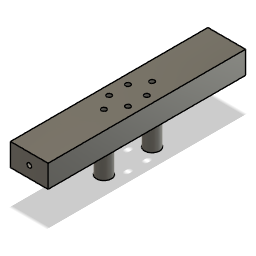
Assemply v7 (Autodesk Fusion 360 archive; units mm, degrees)
design "GPS+hinge stand"
Autodesk Fusion 360 part; units mm, degrees
(part 1 of 5)
sketch "Sketch1" plane through (0, 0, 0) normal (0, 0, 1) x (1, 0, 0)
  line L0 (0, 0) -> (25, 0)
  line L1 (25, 0) -> (25, 15)
  line L2 (25, 15) -> (0, 15)
  line L3 (0, 15) -> (0, 0)
  dimension "d1" = 25
  dimension "d2" = 15
  constraint horizontal L0
  constraint vertical L1
  constraint horizontal L2
  constraint vertical L3
  constraint coincident L0.start L3.end
  measures "d1" distance of L0.start L0.end
  measures "d2" distance of L0.start L2.end
extrude "Extrude1" add sketch "Sketch1" along normal blind 131.11
sketch "Sketch2" plane through (0, 0, 131.11) normal (0, 0, 1) x (1, 0, 0)
  line L0 (0, 15) -> (0, 0)
  line L1 (0, 0) -> (25, 0)
  line L2 (25, 0) -> (25, 15)
  line L3 (25, 15) -> (0, 15)
  circle A0 centre (12.5, 7.5) radius 1.5
  dimension "d5" = 3
  measures "d5" diameter of A0
extrude "Extrude2" cut sketch "Sketch2" against normal blind 180 contours A0
sketch "Sketch3" plane through (0, 15, 0) normal (0, 1, 0) x (-1, 0, 0)
  line L0 (-25, 0) -> (0, 0)
  line L1 (0, 0) -> (0, 131.11)
  line L2 (0, 131.11) -> (-25, 131.11)
  line L3 (-25, 131.11) -> (-25, 0)
  circle A0 centre (-12.5, 49.555) radius 1.6
  circle A1 centre (-12.5, 81.555) radius 1.6
  dimension "d8" = 3.2
  dimension "d24" = 3.2
  measures "d8" diameter of A0
  measures "d24" diameter of A1
extrude "Extrude3" cut sketch "Sketch3" against normal blind 51 contours A0 | A1
sketch "Sketch4" plane through (0, 15, 0) normal (0, 1, 0) x (-1, 0, 0)
  circle A0 centre (-12.5, 81.555) radius 1.6
  circle A1 centre (-12.5, 49.555) radius 1.6
  line L0 (-25, 0) -> (0, 0)
  line L1 (0, 0) -> (0, 131.11)
  line L2 (0, 131.11) -> (-25, 131.11)
  line L3 (-25, 131.11) -> (-25, 0)
  line L4 (-25, 78.055) -> (0, 78.055)
  line L5 (0, 78.055) -> (0, 53.055)
  line L6 (0, 53.055) -> (-25, 53.055)
  line L7 (-25, 53.055) -> (-25, 78.055)
  line L8 (-25, 78.055) -> (0, 53.055) construction
  line L9 (0, 78.055) -> (-25, 53.055) construction
  point P0 (-12.5, 65.555)
  dimension "d12" = 25
  dimension "d13" = 25
  constraint horizontal L4
  constraint perpendicular L4 L5
  constraint parallel L4 L6
  constraint parallel L5 L7
  constraint coincident L8 P0
  constraint coincident L9 P0
  measures "d12" distance of L5.end L6.end
  measures "d13" distance of L4.end L5.end
sketch "Sketch6" plane through (0, 0, 0) normal (0, -1, 0) x (1, 0, 0)
  circle A0 centre (12.5, 81.555) radius 1.6
  circle A1 centre (12.5, 49.555) radius 1.6
  line L0 (0, 0) -> (25, 0)
  line L1 (25, 0) -> (25, 131.11)
  line L2 (25, 131.11) -> (0, 131.11)
  line L3 (0, 131.11) -> (0, 0)
  circle A2 centre (12.5, 81.555) radius 5
  circle A3 centre (12.5, 49.555) radius 5
  dimension "d20" = 10
  dimension "d21" = 10
  constraint concentric A0 A2
  constraint concentric A1 A3
  measures "d20" diameter of A2
  measures "d21" diameter of A3
extrude "Extrude6" add sketch "Sketch6" along normal blind 22.5 contours A2 | A3
sketch "Sketch7" plane through (0, 15, 0) normal (0, 1, 0) x (-1, 0, 0)
  circle A0 centre (-12.5, 81.555) radius 1.6
  circle A1 centre (-12.5, 49.555) radius 1.6
  line L0 (-25, 0) -> (0, 0)
  line L1 (0, 0) -> (0, 131.11)
  line L2 (0, 131.11) -> (-25, 131.11)
  line L3 (-25, 131.11) -> (-25, 0)
  line L4 (-25, 53.055) -> (0, 53.055)
  line L5 (0, 53.055) -> (0, 78.055)
  line L6 (0, 78.055) -> (-25, 78.055)
  line L7 (-25, 78.055) -> (-25, 53.055)
  circle A2 centre (-6.25, 59.305) radius 1.6
  circle A3 centre (-6.25, 71.805) radius 1.6
  line L8 (-12.5, 65.555) -> (-12.5, 69)
  circle A4 centre (-18.75, 59.305) radius 1.6
  circle A5 centre (-18.75, 71.805) radius 1.6
  point P0 (-12.5, 65.555)
  dimension "d25" = 25
  dimension "d26" = 25
  dimension "d27" = 3.2
  dimension "d28" = 6.25
  dimension "d29" = 6.25
  dimension "d30" = 3.2
  dimension "d31" = 12.5
  constraint horizontal L4
  constraint perpendicular L4 L5
  constraint parallel L4 L6
  constraint parallel L5 L7
  constraint coincident P0 L8.start
  constraint parallel L5 L8
  constraint symmetric A2 L8 A4
  constraint symmetric A3 L8 A5
  measures "d25" distance of L5.end L6.end
  measures "d26" distance of L4.end L5.end
  measures "d27" diameter of A2
  measures "d28" horizontal distance of P0 A2.centre
  measures "d29" distance of L4 A2.centre
  measures "d30" diameter of A3
  measures "d31" distance of A2.centre A3.centre
extrude "Extrude7" cut sketch "Sketch7" against normal blind 17 contours A2 | A3 | A4 | A5
fillet "Fillet1" radius 7.5 2 edges at (7.8384, 0, 83.3631) (7.8384, 0, 51.3631)
sketch "Sketch8" plane through (0, 0, 0) normal (0, -1, 0) x (1, 0, 0)
  arc A0 (4.6502, 59.2828) -> (0, 49.555) centre (12.5, 49.555) ccw
  arc A1 (6.9381, 60.7495) -> (4.6502, 59.2828) centre (6.25, 59.305) ccw
  arc A2 (18.0619, 60.7495) -> (6.9381, 60.7495) centre (12.5, 49.555) ccw
  arc A3 (20.3498, 59.2828) -> (18.0619, 60.7495) centre (18.75, 59.305) ccw
  arc A4 (25, 49.555) -> (20.3498, 59.2828) centre (12.5, 49.555) ccw
  line L0 (25, 49.555) -> (25, 81.555)
  arc A5 (20.3498, 71.8272) -> (25, 81.555) centre (12.5, 81.555) ccw
  arc A6 (18.0619, 70.3605) -> (20.3498, 71.8272) centre (18.75, 71.805) ccw
  arc A7 (6.9381, 70.3605) -> (18.0619, 70.3605) centre (12.5, 81.555) ccw
  arc A8 (4.6502, 71.8272) -> (6.9381, 70.3605) centre (6.25, 71.805) ccw
  arc A9 (0, 81.555) -> (4.6502, 71.8272) centre (12.5, 81.555) ccw
  line L1 (0, 81.555) -> (0, 49.555)
  circle A10 centre (6.25, 59.305) radius 3.5
  circle A11 centre (18.75, 59.305) radius 3.5
  circle A12 centre (6.25, 71.805) radius 3.5
  circle A13 centre (18.75, 71.805) radius 3.5
  dimension "d36" = 7
  dimension "d37" = 7
  dimension "d38" = 7
  dimension "d39" = 7
  constraint concentric A1 A10
  constraint concentric A3 A11
  constraint concentric A8 A12
  constraint concentric A6 A13
  measures "d36" diameter of A10
  measures "d37" diameter of A11
  measures "d38" diameter of A12
  measures "d39" diameter of A13
extrude "Extrude8" cut sketch "Sketch8" along normal blind 6 contours A0 A1 A2 A10 | A2 A3 A4 A11 | A7 A8 A9 A12 | A5 A6 A7 A13 picked at (6.5291, 58.7685) picked at (18.3538, 58.8458) picked at (6.5291, 72.3415) picked at (18.4982, 72.3568)
equation "d22 = 42.5 mm - 40 mm + 20 mm"
equation "d28 = 25 / 4 * 1 mm"
equation "d31 = 25 / 2 * 1 mm"

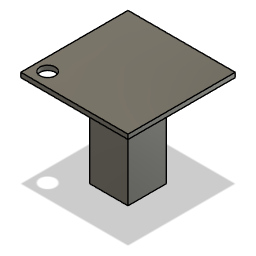
design "Gps mount"
Autodesk Fusion 360 part; units mm, degrees
sketch "Sketch1" plane through (0, 0, 0) normal (0, 1, 0) x (1, 0, 0)
  line L0 (0, 0) -> (25, 0)
  line L1 (25, 0) -> (25, -25)
  line L2 (25, -25) -> (0, -25)
  line L3 (0, -25) -> (0, 0)
  dimension "d1" = 25
  dimension "d2" = 25
  constraint horizontal L0
  constraint vertical L1
  constraint horizontal L2
  constraint vertical L3
  constraint coincident L0.start L3.end
  measures "d1" distance of L0.start L0.end
  measures "d2" distance of L0.start L2.end
extrude "Extrude1" add sketch "Sketch1" along normal blind 60
sketch "Sketch2" plane through (0, 60, 0) normal (0, 1, 0) x (-1, 0, 0)
  line L0 (0, 25) -> (-25, 25)
  line L1 (-25, 25) -> (-25, 0)
  line L2 (-25, 0) -> (0, 0)
  line L3 (0, 0) -> (0, 25)
  line L4 (-47.5, 47.5) -> (22.5, 47.5)
  line L5 (22.5, 47.5) -> (22.5, -22.5)
  line L6 (22.5, -22.5) -> (-47.5, -22.5)
  line L7 (-47.5, -22.5) -> (-47.5, 47.5)
  line L8 (-47.5, 47.5) -> (22.5, -22.5) construction
  line L9 (22.5, 47.5) -> (-47.5, -22.5) construction
  point P0 (-12.5, 12.5)
  dimension "d5" = 70
  dimension "d6" = 70
  constraint horizontal L4
  constraint perpendicular L4 L5
  constraint parallel L4 L6
  constraint parallel L5 L7
  constraint coincident L8 P0
  constraint coincident L9 P0
  measures "d5" distance of L5.end L6.end
  measures "d6" distance of L4.end L5.end
extrude "Extrude2" add sketch "Sketch2" along normal blind 3 contours L0 L1 L2 L3 | L4 L5 L6 L7
fillet "Fillet1" radius 10 4 edges at (12.5, 60, 25) (25, 60, 12.5) (0, 60, 12.5) (12.5, 60, 0)
sketch "Sketch3" plane through (0, 63, 0) normal (0, 1, 0) x (-1, 0, 0)
  line L0 (-47.5, -22.5) -> (22.5, -22.5)
  line L1 (22.5, -22.5) -> (22.5, 47.5)
  line L2 (22.5, 47.5) -> (-47.5, 47.5)
  line L3 (-47.5, 47.5) -> (-47.5, -22.5)
  circle A0 centre (14.2428, 38.2388) radius 5
  dimension "d11" = 10
  measures "d11" diameter of A0
extrude "Extrude3" cut sketch "Sketch3" against normal blind 30 contours A0
sketch "Sketch4" plane through (0, 0, 0) normal (0, 1, 0) x (1, 0, 0)
  line L0 (25, 0) -> (0, 0)
  line L1 (0, 0) -> (0, -25)
  line L2 (0, -25) -> (25, -25)
  line L3 (25, -25) -> (25, 0)
  circle A0 centre (18.75, -6.25) radius 1.5
  circle A1 centre (18.767, -18.75) radius 1.5
  circle A2 centre (6.25, -6.25) radius 1.5
  circle A3 centre (6.233, -18.75) radius 1.5
  point P0 (25, 0)
  point P1 (25, -25)
  dimension "d14" = 3
  dimension "d15" = 3
  dimension "d17" = 12.5
  dimension "d18" = 6.25
  constraint horizontal L0
  constraint vertical L1
  constraint horizontal L2
  constraint vertical L3
  constraint coincident L0 P0
  constraint coincident L2 P1
  measures "d14" diameter of A0
  measures "d15" diameter of A1
  measures "d17" vertical distance of A0.centre A1.centre
  measures "d18" distance of L2 A1.centre
extrude "Extrude4" cut sketch "Sketch4" along normal blind 7 contours A0 | A1 | A2 | A3
equation "d17 = 2.5 / 2 * 1 cm"
equation "d18 = 2.5 / 4 * 1 cm"

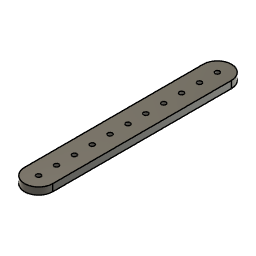
design "Camera arm 1"
Autodesk Fusion 360 part; units mm, degrees
sketch "Sketch1" plane through (0, 0, 0) normal (0, 1, 0) x (1, 0, 0)
  line L0 (20, 0) -> (20, -127)
  line L1 (0, -127) -> (0, 0)
  arc A0 (0, -127) -> (20, -127) centre (10, -127) ccw
  arc A1 (20, 0) -> (0, 0) centre (10, 0) ccw
  circle A2 centre (10, 0) radius 1.6
  circle A3 centre (10, -127) radius 1.6
  circle A4 centre (10, -114.3) radius 1.6
  circle A5 centre (10, -101.6) radius 1.6
  circle A6 centre (10, -88.9) radius 1.6
  circle A7 centre (10, -76.2) radius 1.6
  circle A8 centre (10, -63.5) radius 1.6
  circle A9 centre (10, -50.8) radius 1.6
  circle A10 centre (10, -38.1) radius 1.6
  circle A11 centre (10, -25.4) radius 1.6
  circle A12 centre (10, -12.7) radius 1.6
  dimension "d1" = 20
  dimension "d2" = 127
  dimension "d3" = 3.2
  dimension "d4" = 3.2
  dimension "d9" = 0
  dimension "d10" = 12.7
  constraint vertical L0
  constraint vertical L1
  constraint coincident L1.end A1.end
  constraint concentric A1 A2
  constraint concentric A0 A3
  measures "d1" distance of L1.end L0.start
  measures "d2" distance of L1.end L1.start
  measures "d3" diameter of A2
  measures "d4" diameter of A3
extrude "Extrude1" add sketch "Sketch1" along normal blind 5

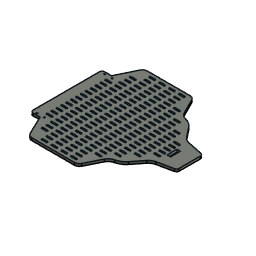
design "Electronics plate"
Autodesk Fusion 360 part; units mm, degrees
sketch "Sketch2" plane through (0, 0, 0) normal (0, 1, 0) x (1, 0, 0)
  line L0 (-228.4396, 191.0218) -> (-250, 146.0218)
  line L1 (-249.9865, 0) -> (-228.4396, -44.9718)
  line L2 (-128.4396, 191.0218) -> (-228.4396, 191.0218)
  line L3 (-228.4396, -44.9718) -> (-128.4396, -44.9718)
  line L4 (-105.9194, 146.05) -> (-128.4396, 191.0218)
  line L5 (-128.4396, -44.9718) -> (-105.9194, 0)
  line L6 (-138.6977, 71.525) -> (-143.6977, 71.525)
  line L7 (-148.6977, 74.525) -> (-138.6977, 74.525)
  arc A0 (-138.6977, 71.525) -> (-138.6977, 74.525) centre (-138.6977, 73.025) ccw
  arc A1 (-148.6977, 74.525) -> (-148.6977, 71.525) centre (-148.6977, 73.025) ccw
  line L8 (-148.6977, 71.525) -> (-143.6977, 71.525)
  arc A2 (-208.6977, -35.475) -> (-208.6977, -38.475) centre (-208.6977, -36.975) ccw
  arc A3 (-198.6977, -38.475) -> (-198.6977, -35.475) centre (-198.6977, -36.975) ccw
  line L9 (-208.6977, -35.475) -> (-198.6977, -35.475)
  line L10 (-208.6977, -38.475) -> (-203.6977, -38.475)
  line L11 (-198.6977, -38.475) -> (-203.6977, -38.475)
  arc A4 (-188.6977, -35.475) -> (-188.6977, -38.475) centre (-188.6977, -36.975) ccw
  arc A5 (-178.6977, -38.475) -> (-178.6977, -35.475) centre (-178.6977, -36.975) ccw
  line L12 (-188.6977, -35.475) -> (-178.6977, -35.475)
  line L13 (-188.6977, -38.475) -> (-183.6977, -38.475)
  line L14 (-178.6977, -38.475) -> (-183.6977, -38.475)
  arc A6 (-168.6977, -35.475) -> (-168.6977, -38.475) centre (-168.6977, -36.975) ccw
  arc A7 (-158.6977, -38.475) -> (-158.6977, -35.475) centre (-158.6977, -36.975) ccw
  line L15 (-168.6977, -35.475) -> (-158.6977, -35.475)
  line L16 (-168.6977, -38.475) -> (-163.6977, -38.475)
  line L17 (-158.6977, -38.475) -> (-163.6977, -38.475)
  arc A8 (-148.6977, -35.475) -> (-148.6977, -38.475) centre (-148.6977, -36.975) ccw
  arc A9 (-138.6977, -38.475) -> (-138.6977, -35.475) centre (-138.6977, -36.975) ccw
  line L18 (-148.6977, -35.475) -> (-138.6977, -35.475)
  line L19 (-148.6977, -38.475) -> (-143.6977, -38.475)
  line L20 (-138.6977, -38.475) -> (-143.6977, -38.475)
  arc A10 (-208.6977, -25.475) -> (-208.6977, -28.475) centre (-208.6977, -26.975) ccw
  arc A11 (-198.6977, -28.475) -> (-198.6977, -25.475) centre (-198.6977, -26.975) ccw
  line L21 (-208.6977, -25.475) -> (-198.6977, -25.475)
  line L22 (-208.6977, -28.475) -> (-203.6977, -28.475)
  line L23 (-198.6977, -28.475) -> (-203.6977, -28.475)
  arc A12 (-188.6977, -25.475) -> (-188.6977, -28.475) centre (-188.6977, -26.975) ccw
  arc A13 (-178.6977, -28.475) -> (-178.6977, -25.475) centre (-178.6977, -26.975) ccw
  line L24 (-188.6977, -25.475) -> (-178.6977, -25.475)
  line L25 (-188.6977, -28.475) -> (-183.6977, -28.475)
  line L26 (-178.6977, -28.475) -> (-183.6977, -28.475)
  arc A14 (-168.6977, -25.475) -> (-168.6977, -28.475) centre (-168.6977, -26.975) ccw
  arc A15 (-158.6977, -28.475) -> (-158.6977, -25.475) centre (-158.6977, -26.975) ccw
  line L27 (-168.6977, -25.475) -> (-158.6977, -25.475)
  line L28 (-168.6977, -28.475) -> (-163.6977, -28.475)
  line L29 (-158.6977, -28.475) -> (-163.6977, -28.475)
  arc A16 (-148.6977, -25.475) -> (-148.6977, -28.475) centre (-148.6977, -26.975) ccw
  arc A17 (-138.6977, -28.475) -> (-138.6977, -25.475) centre (-138.6977, -26.975) ccw
  line L30 (-148.6977, -25.475) -> (-138.6977, -25.475)
  line L31 (-148.6977, -28.475) -> (-143.6977, -28.475)
  line L32 (-138.6977, -28.475) -> (-143.6977, -28.475)
  arc A18 (-228.6977, -15.475) -> (-228.6977, -18.475) centre (-228.6977, -16.975) ccw
  arc A19 (-218.6977, -18.475) -> (-218.6977, -15.475) centre (-218.6977, -16.975) ccw
  line L33 (-228.6977, -15.475) -> (-218.6977, -15.475)
  line L34 (-228.6977, -18.475) -> (-223.6977, -18.475)
  line L35 (-218.6977, -18.475) -> (-223.6977, -18.475)
  arc A20 (-208.6977, -15.475) -> (-208.6977, -18.475) centre (-208.6977, -16.975) ccw
  arc A21 (-198.6977, -18.475) -> (-198.6977, -15.475) centre (-198.6977, -16.975) ccw
  line L36 (-208.6977, -15.475) -> (-198.6977, -15.475)
  line L37 (-208.6977, -18.475) -> (-203.6977, -18.475)
  line L38 (-198.6977, -18.475) -> (-203.6977, -18.475)
  arc A22 (-188.6977, -15.475) -> (-188.6977, -18.475) centre (-188.6977, -16.975) ccw
  arc A23 (-178.6977, -18.475) -> (-178.6977, -15.475) centre (-178.6977, -16.975) ccw
  line L39 (-188.6977, -15.475) -> (-178.6977, -15.475)
  line L40 (-188.6977, -18.475) -> (-183.6977, -18.475)
  line L41 (-178.6977, -18.475) -> (-183.6977, -18.475)
  arc A24 (-168.6977, -15.475) -> (-168.6977, -18.475) centre (-168.6977, -16.975) ccw
  arc A25 (-158.6977, -18.475) -> (-158.6977, -15.475) centre (-158.6977, -16.975) ccw
  line L42 (-168.6977, -15.475) -> (-158.6977, -15.475)
  line L43 (-168.6977, -18.475) -> (-163.6977, -18.475)
  line L44 (-158.6977, -18.475) -> (-163.6977, -18.475)
  arc A26 (-148.6977, -15.475) -> (-148.6977, -18.475) centre (-148.6977, -16.975) ccw
  arc A27 (-138.6977, -18.475) -> (-138.6977, -15.475) centre (-138.6977, -16.975) ccw
  line L45 (-148.6977, -15.475) -> (-138.6977, -15.475)
  line L46 (-148.6977, -18.475) -> (-143.6977, -18.475)
  line L47 (-138.6977, -18.475) -> (-143.6977, -18.475)
  arc A28 (-228.6977, -5.475) -> (-228.6977, -8.475) centre (-228.6977, -6.975) ccw
  arc A29 (-218.6977, -8.475) -> (-218.6977, -5.475) centre (-218.6977, -6.975) ccw
  line L48 (-228.6977, -5.475) -> (-218.6977, -5.475)
  line L49 (-228.6977, -8.475) -> (-223.6977, -8.475)
  line L50 (-218.6977, -8.475) -> (-223.6977, -8.475)
  arc A30 (-208.6977, -5.475) -> (-208.6977, -8.475) centre (-208.6977, -6.975) ccw
  arc A31 (-198.6977, -8.475) -> (-198.6977, -5.475) centre (-198.6977, -6.975) ccw
  line L51 (-208.6977, -5.475) -> (-198.6977, -5.475)
  line L52 (-208.6977, -8.475) -> (-203.6977, -8.475)
  line L53 (-198.6977, -8.475) -> (-203.6977, -8.475)
  arc A32 (-188.6977, -5.475) -> (-188.6977, -8.475) centre (-188.6977, -6.975) ccw
  arc A33 (-178.6977, -8.475) -> (-178.6977, -5.475) centre (-178.6977, -6.975) ccw
  line L54 (-188.6977, -5.475) -> (-178.6977, -5.475)
  line L55 (-188.6977, -8.475) -> (-183.6977, -8.475)
  line L56 (-178.6977, -8.475) -> (-183.6977, -8.475)
  arc A34 (-168.6977, -5.475) -> (-168.6977, -8.475) centre (-168.6977, -6.975) ccw
  arc A35 (-158.6977, -8.475) -> (-158.6977, -5.475) centre (-158.6977, -6.975) ccw
  line L57 (-168.6977, -5.475) -> (-158.6977, -5.475)
  line L58 (-168.6977, -8.475) -> (-163.6977, -8.475)
  line L59 (-158.6977, -8.475) -> (-163.6977, -8.475)
  arc A36 (-148.6977, -5.475) -> (-148.6977, -8.475) centre (-148.6977, -6.975) ccw
  arc A37 (-138.6977, -8.475) -> (-138.6977, -5.475) centre (-138.6977, -6.975) ccw
  line L60 (-148.6977, -5.475) -> (-138.6977, -5.475)
  line L61 (-148.6977, -8.475) -> (-143.6977, -8.475)
  line L62 (-138.6977, -8.475) -> (-143.6977, -8.475)
  arc A38 (-128.6977, -5.475) -> (-128.6977, -8.475) centre (-128.6977, -6.975) ccw
  arc A39 (-118.6977, -8.475) -> (-118.6977, -5.475) centre (-118.6977, -6.975) ccw
  line L63 (-128.6977, -5.475) -> (-118.6977, -5.475)
  line L64 (-128.6977, -8.475) -> (-123.6977, -8.475)
  line L65 (-118.6977, -8.475) -> (-123.6977, -8.475)
  arc A40 (-228.6977, 4.525) -> (-228.6977, 1.525) centre (-228.6977, 3.025) ccw
  arc A41 (-218.6977, 1.525) -> (-218.6977, 4.525) centre (-218.6977, 3.025) ccw
  line L66 (-228.6977, 4.525) -> (-218.6977, 4.525)
  line L67 (-228.6977, 1.525) -> (-223.6977, 1.525)
  line L68 (-218.6977, 1.525) -> (-223.6977, 1.525)
  arc A42 (-208.6977, 4.525) -> (-208.6977, 1.525) centre (-208.6977, 3.025) ccw
  arc A43 (-198.6977, 1.525) -> (-198.6977, 4.525) centre (-198.6977, 3.025) ccw
  line L69 (-208.6977, 4.525) -> (-198.6977, 4.525)
  line L70 (-208.6977, 1.525) -> (-203.6977, 1.525)
  line L71 (-198.6977, 1.525) -> (-203.6977, 1.525)
  arc A44 (-188.6977, 4.525) -> (-188.6977, 1.525) centre (-188.6977, 3.025) ccw
  arc A45 (-178.6977, 1.525) -> (-178.6977, 4.525) centre (-178.6977, 3.025) ccw
  line L72 (-188.6977, 4.525) -> (-178.6977, 4.525)
  line L73 (-188.6977, 1.525) -> (-183.6977, 1.525)
  line L74 (-178.6977, 1.525) -> (-183.6977, 1.525)
  arc A46 (-168.6977, 4.525) -> (-168.6977, 1.525) centre (-168.6977, 3.025) ccw
  arc A47 (-158.6977, 1.525) -> (-158.6977, 4.525) centre (-158.6977, 3.025) ccw
  line L75 (-168.6977, 4.525) -> (-158.6977, 4.525)
  line L76 (-168.6977, 1.525) -> (-163.6977, 1.525)
  line L77 (-158.6977, 1.525) -> (-163.6977, 1.525)
  arc A48 (-148.6977, 4.525) -> (-148.6977, 1.525) centre (-148.6977, 3.025) ccw
  arc A49 (-138.6977, 1.525) -> (-138.6977, 4.525) centre (-138.6977, 3.025) ccw
  line L78 (-148.6977, 4.525) -> (-138.6977, 4.525)
  line L79 (-148.6977, 1.525) -> (-143.6977, 1.525)
  line L80 (-138.6977, 1.525) -> (-143.6977, 1.525)
  arc A50 (-128.6977, 4.525) -> (-128.6977, 1.525) centre (-128.6977, 3.025) ccw
  arc A51 (-118.6977, 1.525) -> (-118.6977, 4.525) centre (-118.6977, 3.025) ccw
  line L81 (-128.6977, 4.525) -> (-118.6977, 4.525)
  line L82 (-128.6977, 1.525) -> (-123.6977, 1.525)
  line L83 (-118.6977, 1.525) -> (-123.6977, 1.525)
  arc A52 (-248.6977, 14.525) -> (-248.6977, 11.525) centre (-248.6977, 13.025) ccw
  arc A53 (-238.6977, 11.525) -> (-238.6977, 14.525) centre (-238.6977, 13.025) ccw
  line L84 (-248.6977, 14.525) -> (-238.6977, 14.525)
  line L85 (-248.6977, 11.525) -> (-243.6977, 11.525)
  line L86 (-238.6977, 11.525) -> (-243.6977, 11.525)
  arc A54 (-228.6977, 14.525) -> (-228.6977, 11.525) centre (-228.6977, 13.025) ccw
  arc A55 (-218.6977, 11.525) -> (-218.6977, 14.525) centre (-218.6977, 13.025) ccw
  line L87 (-228.6977, 14.525) -> (-218.6977, 14.525)
  line L88 (-228.6977, 11.525) -> (-223.6977, 11.525)
  line L89 (-218.6977, 11.525) -> (-223.6977, 11.525)
  arc A56 (-208.6977, 14.525) -> (-208.6977, 11.525) centre (-208.6977, 13.025) ccw
  arc A57 (-198.6977, 11.525) -> (-198.6977, 14.525) centre (-198.6977, 13.025) ccw
  line L90 (-208.6977, 14.525) -> (-198.6977, 14.525)
  line L91 (-208.6977, 11.525) -> (-203.6977, 11.525)
  line L92 (-198.6977, 11.525) -> (-203.6977, 11.525)
  arc A58 (-188.6977, 14.525) -> (-188.6977, 11.525) centre (-188.6977, 13.025) ccw
  arc A59 (-178.6977, 11.525) -> (-178.6977, 14.525) centre (-178.6977, 13.025) ccw
  line L93 (-188.6977, 14.525) -> (-178.6977, 14.525)
  line L94 (-188.6977, 11.525) -> (-183.6977, 11.525)
  line L95 (-178.6977, 11.525) -> (-183.6977, 11.525)
  arc A60 (-168.6977, 14.525) -> (-168.6977, 11.525) centre (-168.6977, 13.025) ccw
  arc A61 (-158.6977, 11.525) -> (-158.6977, 14.525) centre (-158.6977, 13.025) ccw
  line L96 (-168.6977, 14.525) -> (-158.6977, 14.525)
  line L97 (-168.6977, 11.525) -> (-163.6977, 11.525)
  line L98 (-158.6977, 11.525) -> (-163.6977, 11.525)
  arc A62 (-148.6977, 14.525) -> (-148.6977, 11.525) centre (-148.6977, 13.025) ccw
  arc A63 (-138.6977, 11.525) -> (-138.6977, 14.525) centre (-138.6977, 13.025) ccw
  line L99 (-148.6977, 14.525) -> (-138.6977, 14.525)
  line L100 (-148.6977, 11.525) -> (-143.6977, 11.525)
  line L101 (-138.6977, 11.525) -> (-143.6977, 11.525)
  arc A64 (-128.6977, 14.525) -> (-128.6977, 11.525) centre (-128.6977, 13.025) ccw
  arc A65 (-118.6977, 11.525) -> (-118.6977, 14.525) centre (-118.6977, 13.025) ccw
  line L102 (-128.6977, 14.525) -> (-118.6977, 14.525)
  line L103 (-128.6977, 11.525) -> (-123.6977, 11.525)
  line L104 (-118.6977, 11.525) -> (-123.6977, 11.525)
  arc A66 (-108.6977, 14.525) -> (-108.6977, 11.525) centre (-108.6977, 13.025) ccw
  arc A67 (-98.6977, 11.525) -> (-98.6977, 14.525) centre (-98.6977, 13.025) ccw
  line L105 (-108.6977, 14.525) -> (-98.6977, 14.525)
  line L106 (-108.6977, 11.525) -> (-103.6977, 11.525)
  line L107 (-98.6977, 11.525) -> (-103.6977, 11.525)
  arc A68 (-248.6977, 24.525) -> (-248.6977, 21.525) centre (-248.6977, 23.025) ccw
  arc A69 (-238.6977, 21.525) -> (-238.6977, 24.525) centre (-238.6977, 23.025) ccw
  line L108 (-248.6977, 24.525) -> (-238.6977, 24.525)
  line L109 (-248.6977, 21.525) -> (-243.6977, 21.525)
  line L110 (-238.6977, 21.525) -> (-243.6977, 21.525)
  arc A70 (-228.6977, 24.525) -> (-228.6977, 21.525) centre (-228.6977, 23.025) ccw
  arc A71 (-218.6977, 21.525) -> (-218.6977, 24.525) centre (-218.6977, 23.025) ccw
  line L111 (-228.6977, 24.525) -> (-218.6977, 24.525)
  line L112 (-228.6977, 21.525) -> (-223.6977, 21.525)
  line L113 (-218.6977, 21.525) -> (-223.6977, 21.525)
  arc A72 (-208.6977, 24.525) -> (-208.6977, 21.525) centre (-208.6977, 23.025) ccw
  arc A73 (-198.6977, 21.525) -> (-198.6977, 24.525) centre (-198.6977, 23.025) ccw
  line L114 (-208.6977, 24.525) -> (-198.6977, 24.525)
  line L115 (-208.6977, 21.525) -> (-203.6977, 21.525)
  line L116 (-198.6977, 21.525) -> (-203.6977, 21.525)
  arc A74 (-188.6977, 24.525) -> (-188.6977, 21.525) centre (-188.6977, 23.025) ccw
  arc A75 (-178.6977, 21.525) -> (-178.6977, 24.525) centre (-178.6977, 23.025) ccw
  line L117 (-188.6977, 24.525) -> (-178.6977, 24.525)
  line L118 (-188.6977, 21.525) -> (-183.6977, 21.525)
  line L119 (-178.6977, 21.525) -> (-183.6977, 21.525)
  arc A76 (-168.6977, 24.525) -> (-168.6977, 21.525) centre (-168.6977, 23.025) ccw
  arc A77 (-158.6977, 21.525) -> (-158.6977, 24.525) centre (-158.6977, 23.025) ccw
  line L120 (-168.6977, 24.525) -> (-158.6977, 24.525)
  line L121 (-168.6977, 21.525) -> (-163.6977, 21.525)
  line L122 (-158.6977, 21.525) -> (-163.6977, 21.525)
  arc A78 (-148.6977, 24.525) -> (-148.6977, 21.525) centre (-148.6977, 23.025) ccw
  arc A79 (-138.6977, 21.525) -> (-138.6977, 24.525) centre (-138.6977, 23.025) ccw
  line L123 (-148.6977, 24.525) -> (-138.6977, 24.525)
  line L124 (-148.6977, 21.525) -> (-143.6977, 21.525)
  line L125 (-138.6977, 21.525) -> (-143.6977, 21.525)
  arc A80 (-128.6977, 24.525) -> (-128.6977, 21.525) centre (-128.6977, 23.025) ccw
  arc A81 (-118.6977, 21.525) -> (-118.6977, 24.525) centre (-118.6977, 23.025) ccw
  line L126 (-128.6977, 24.525) -> (-118.6977, 24.525)
  line L127 (-128.6977, 21.525) -> (-123.6977, 21.525)
  line L128 (-118.6977, 21.525) -> (-123.6977, 21.525)
  arc A82 (-108.6977, 24.525) -> (-108.6977, 21.525) centre (-108.6977, 23.025) ccw
  arc A83 (-98.6977, 21.525) -> (-98.6977, 24.525) centre (-98.6977, 23.025) ccw
  line L129 (-108.6977, 24.525) -> (-98.6977, 24.525)
  line L130 (-108.6977, 21.525) -> (-103.6977, 21.525)
  line L131 (-98.6977, 21.525) -> (-103.6977, 21.525)
  arc A84 (-248.6977, 34.525) -> (-248.6977, 31.525) centre (-248.6977, 33.025) ccw
  arc A85 (-238.6977, 31.525) -> (-238.6977, 34.525) centre (-238.6977, 33.025) ccw
  line L132 (-248.6977, 34.525) -> (-238.6977, 34.525)
  line L133 (-248.6977, 31.525) -> (-243.6977, 31.525)
  line L134 (-238.6977, 31.525) -> (-243.6977, 31.525)
  arc A86 (-228.6977, 34.525) -> (-228.6977, 31.525) centre (-228.6977, 33.025) ccw
  arc A87 (-218.6977, 31.525) -> (-218.6977, 34.525) centre (-218.6977, 33.025) ccw
  line L135 (-228.6977, 34.525) -> (-218.6977, 34.525)
  line L136 (-228.6977, 31.525) -> (-223.6977, 31.525)
  line L137 (-218.6977, 31.525) -> (-223.6977, 31.525)
  arc A88 (-208.6977, 34.525) -> (-208.6977, 31.525) centre (-208.6977, 33.025) ccw
  arc A89 (-198.6977, 31.525) -> (-198.6977, 34.525) centre (-198.6977, 33.025) ccw
  line L138 (-208.6977, 34.525) -> (-198.6977, 34.525)
  line L139 (-208.6977, 31.525) -> (-203.6977, 31.525)
  line L140 (-198.6977, 31.525) -> (-203.6977, 31.525)
  arc A90 (-188.6977, 34.525) -> (-188.6977, 31.525) centre (-188.6977, 33.025) ccw
  arc A91 (-178.6977, 31.525) -> (-178.6977, 34.525) centre (-178.6977, 33.025) ccw
  line L141 (-188.6977, 34.525) -> (-178.6977, 34.525)
  line L142 (-188.6977, 31.525) -> (-183.6977, 31.525)
  line L143 (-178.6977, 31.525) -> (-183.6977, 31.525)
  arc A92 (-168.6977, 34.525) -> (-168.6977, 31.525) centre (-168.6977, 33.025) ccw
  arc A93 (-158.6977, 31.525) -> (-158.6977, 34.525) centre (-158.6977, 33.025) ccw
  line L144 (-168.6977, 34.525) -> (-158.6977, 34.525)
  line L145 (-168.6977, 31.525) -> (-163.6977, 31.525)
  line L146 (-158.6977, 31.525) -> (-163.6977, 31.525)
  arc A94 (-148.6977, 34.525) -> (-148.6977, 31.525) centre (-148.6977, 33.025) ccw
  arc A95 (-138.6977, 31.525) -> (-138.6977, 34.525) centre (-138.6977, 33.025) ccw
  line L147 (-148.6977, 34.525) -> (-138.6977, 34.525)
  line L148 (-148.6977, 31.525) -> (-143.6977, 31.525)
  line L149 (-138.6977, 31.525) -> (-143.6977, 31.525)
  arc A96 (-128.6977, 34.525) -> (-128.6977, 31.525) centre (-128.6977, 33.025) ccw
  arc A97 (-118.6977, 31.525) -> (-118.6977, 34.525) centre (-118.6977, 33.025) ccw
  line L150 (-128.6977, 34.525) -> (-118.6977, 34.525)
  line L151 (-128.6977, 31.525) -> (-123.6977, 31.525)
  line L152 (-118.6977, 31.525) -> (-123.6977, 31.525)
  arc A98 (-108.6977, 34.525) -> (-108.6977, 31.525) centre (-108.6977, 33.025) ccw
  arc A99 (-98.6977, 31.525) -> (-98.6977, 34.525) centre (-98.6977, 33.025) ccw
  line L153 (-108.6977, 34.525) -> (-98.6977, 34.525)
  line L154 (-108.6977, 31.525) -> (-103.6977, 31.525)
  line L155 (-98.6977, 31.525) -> (-103.6977, 31.525)
  arc A100 (-88.6977, 34.525) -> (-88.6977, 31.525) centre (-88.6977, 33.025) ccw
  arc A101 (-78.6977, 31.525) -> (-78.6977, 34.525) centre (-78.6977, 33.025) ccw
  line L156 (-88.6977, 34.525) -> (-78.6977, 34.525)
  line L157 (-88.6977, 31.525) -> (-83.6977, 31.525)
  line L158 (-78.6977, 31.525) -> (-83.6977, 31.525)
  arc A102 (-248.6977, 44.525) -> (-248.6977, 41.525) centre (-248.6977, 43.025) ccw
  arc A103 (-238.6977, 41.525) -> (-238.6977, 44.525) centre (-238.6977, 43.025) ccw
  line L159 (-248.6977, 44.525) -> (-238.6977, 44.525)
  line L160 (-248.6977, 41.525) -> (-243.6977, 41.525)
  line L161 (-238.6977, 41.525) -> (-243.6977, 41.525)
  arc A104 (-228.6977, 44.525) -> (-228.6977, 41.525) centre (-228.6977, 43.025) ccw
  arc A105 (-218.6977, 41.525) -> (-218.6977, 44.525) centre (-218.6977, 43.025) ccw
  line L162 (-228.6977, 44.525) -> (-218.6977, 44.525)
  line L163 (-228.6977, 41.525) -> (-223.6977, 41.525)
  line L164 (-218.6977, 41.525) -> (-223.6977, 41.525)
  arc A106 (-208.6977, 44.525) -> (-208.6977, 41.525) centre (-208.6977, 43.025) ccw
  arc A107 (-198.6977, 41.525) -> (-198.6977, 44.525) centre (-198.6977, 43.025) ccw
  line L165 (-208.6977, 44.525) -> (-198.6977, 44.525)
  line L166 (-208.6977, 41.525) -> (-203.6977, 41.525)
  line L167 (-198.6977, 41.525) -> (-203.6977, 41.525)
  arc A108 (-188.6977, 44.525) -> (-188.6977, 41.525) centre (-188.6977, 43.025) ccw
  arc A109 (-178.6977, 41.525) -> (-178.6977, 44.525) centre (-178.6977, 43.025) ccw
  line L168 (-188.6977, 44.525) -> (-178.6977, 44.525)
  line L169 (-188.6977, 41.525) -> (-183.6977, 41.525)
  line L170 (-178.6977, 41.525) -> (-183.6977, 41.525)
  arc A110 (-168.6977, 44.525) -> (-168.6977, 41.525) centre (-168.6977, 43.025) ccw
  arc A111 (-158.6977, 41.525) -> (-158.6977, 44.525) centre (-158.6977, 43.025) ccw
  line L171 (-168.6977, 44.525) -> (-158.6977, 44.525)
  line L172 (-168.6977, 41.525) -> (-163.6977, 41.525)
  line L173 (-158.6977, 41.525) -> (-163.6977, 41.525)
  arc A112 (-148.6977, 44.525) -> (-148.6977, 41.525) centre (-148.6977, 43.025) ccw
  arc A113 (-138.6977, 41.525) -> (-138.6977, 44.525) centre (-138.6977, 43.025) ccw
  line L174 (-148.6977, 44.525) -> (-138.6977, 44.525)
  line L175 (-148.6977, 41.525) -> (-143.6977, 41.525)
  line L176 (-138.6977, 41.525) -> (-143.6977, 41.525)
  arc A114 (-128.6977, 44.525) -> (-128.6977, 41.525) centre (-128.6977, 43.025) ccw
  arc A115 (-118.6977, 41.525) -> (-118.6977, 44.525) centre (-118.6977, 43.025) ccw
  line L177 (-128.6977, 44.525) -> (-118.6977, 44.525)
  line L178 (-128.6977, 41.525) -> (-123.6977, 41.525)
  line L179 (-118.6977, 41.525) -> (-123.6977, 41.525)
  arc A116 (-108.6977, 44.525) -> (-108.6977, 41.525) centre (-108.6977, 43.025) ccw
  arc A117 (-98.6977, 41.525) -> (-98.6977, 44.525) centre (-98.6977, 43.025) ccw
  line L180 (-108.6977, 44.525) -> (-98.6977, 44.525)
  line L181 (-108.6977, 41.525) -> (-103.6977, 41.525)
  line L182 (-98.6977, 41.525) -> (-103.6977, 41.525)
  arc A118 (-88.6977, 44.525) -> (-88.6977, 41.525) centre (-88.6977, 43.025) ccw
  arc A119 (-78.6977, 41.525) -> (-78.6977, 44.525) centre (-78.6977, 43.025) ccw
  line L183 (-88.6977, 44.525) -> (-78.6977, 44.525)
  line L184 (-88.6977, 41.525) -> (-83.6977, 41.525)
  line L185 (-78.6977, 41.525) -> (-83.6977, 41.525)
  arc A120 (-248.6977, 54.525) -> (-248.6977, 51.525) centre (-248.6977, 53.025) ccw
  arc A121 (-238.6977, 51.525) -> (-238.6977, 54.525) centre (-238.6977, 53.025) ccw
  line L186 (-248.6977, 54.525) -> (-238.6977, 54.525)
  line L187 (-248.6977, 51.525) -> (-243.6977, 51.525)
  line L188 (-238.6977, 51.525) -> (-243.6977, 51.525)
  arc A122 (-228.6977, 54.525) -> (-228.6977, 51.525) centre (-228.6977, 53.025) ccw
  arc A123 (-218.6977, 51.525) -> (-218.6977, 54.525) centre (-218.6977, 53.025) ccw
  line L189 (-228.6977, 54.525) -> (-218.6977, 54.525)
  line L190 (-228.6977, 51.525) -> (-223.6977, 51.525)
  line L191 (-218.6977, 51.525) -> (-223.6977, 51.525)
  arc A124 (-208.6977, 54.525) -> (-208.6977, 51.525) centre (-208.6977, 53.025) ccw
  arc A125 (-198.6977, 51.525) -> (-198.6977, 54.525) centre (-198.6977, 53.025) ccw
  line L192 (-208.6977, 54.525) -> (-198.6977, 54.525)
  line L193 (-208.6977, 51.525) -> (-203.6977, 51.525)
  line L194 (-198.6977, 51.525) -> (-203.6977, 51.525)
  arc A126 (-188.6977, 54.525) -> (-188.6977, 51.525) centre (-188.6977, 53.025) ccw
  arc A127 (-178.6977, 51.525) -> (-178.6977, 54.525) centre (-178.6977, 53.025) ccw
  line L195 (-188.6977, 54.525) -> (-178.6977, 54.525)
  line L196 (-188.6977, 51.525) -> (-183.6977, 51.525)
  line L197 (-178.6977, 51.525) -> (-183.6977, 51.525)
  arc A128 (-168.6977, 54.525) -> (-168.6977, 51.525) centre (-168.6977, 53.025) ccw
  arc A129 (-158.6977, 51.525) -> (-158.6977, 54.525) centre (-158.6977, 53.025) ccw
  line L198 (-168.6977, 54.525) -> (-158.6977, 54.525)
  line L199 (-168.6977, 51.525) -> (-163.6977, 51.525)
  line L200 (-158.6977, 51.525) -> (-163.6977, 51.525)
  arc A130 (-148.6977, 54.525) -> (-148.6977, 51.525) centre (-148.6977, 53.025) ccw
  arc A131 (-138.6977, 51.525) -> (-138.6977, 54.525) centre (-138.6977, 53.025) ccw
  line L201 (-148.6977, 54.525) -> (-138.6977, 54.525)
  line L202 (-148.6977, 51.525) -> (-143.6977, 51.525)
  line L203 (-138.6977, 51.525) -> (-143.6977, 51.525)
  arc A132 (-128.6977, 54.525) -> (-128.6977, 51.525) centre (-128.6977, 53.025) ccw
  arc A133 (-118.6977, 51.525) -> (-118.6977, 54.525) centre (-118.6977, 53.025) ccw
  line L204 (-128.6977, 54.525) -> (-118.6977, 54.525)
  line L205 (-128.6977, 51.525) -> (-123.6977, 51.525)
  line L206 (-118.6977, 51.525) -> (-123.6977, 51.525)
  arc A134 (-108.6977, 54.525) -> (-108.6977, 51.525) centre (-108.6977, 53.025) ccw
  arc A135 (-98.6977, 51.525) -> (-98.6977, 54.525) centre (-98.6977, 53.025) ccw
  line L207 (-108.6977, 54.525) -> (-98.6977, 54.525)
  line L208 (-108.6977, 51.525) -> (-103.6977, 51.525)
  line L209 (-98.6977, 51.525) -> (-103.6977, 51.525)
  arc A136 (-88.6977, 54.525) -> (-88.6977, 51.525) centre (-88.6977, 53.025) ccw
  arc A137 (-78.6977, 51.525) -> (-78.6977, 54.525) centre (-78.6977, 53.025) ccw
  line L210 (-88.6977, 54.525) -> (-78.6977, 54.525)
  line L211 (-88.6977, 51.525) -> (-83.6977, 51.525)
  line L212 (-78.6977, 51.525) -> (-83.6977, 51.525)
  arc A138 (-68.6977, 54.525) -> (-68.6977, 51.525) centre (-68.6977, 53.025) ccw
  arc A139 (-58.6977, 51.525) -> (-58.6977, 54.525) centre (-58.6977, 53.025) ccw
  line L213 (-68.6977, 54.525) -> (-58.6977, 54.525)
  line L214 (-68.6977, 51.525) -> (-63.6977, 51.525)
  line L215 (-58.6977, 51.525) -> (-63.6977, 51.525)
  arc A140 (-248.6977, 64.525) -> (-248.6977, 61.525) centre (-248.6977, 63.025) ccw
  arc A141 (-238.6977, 61.525) -> (-238.6977, 64.525) centre (-238.6977, 63.025) ccw
  line L216 (-248.6977, 64.525) -> (-238.6977, 64.525)
  line L217 (-248.6977, 61.525) -> (-243.6977, 61.525)
  line L218 (-238.6977, 61.525) -> (-243.6977, 61.525)
  arc A142 (-228.6977, 64.525) -> (-228.6977, 61.525) centre (-228.6977, 63.025) ccw
  arc A143 (-218.6977, 61.525) -> (-218.6977, 64.525) centre (-218.6977, 63.025) ccw
  line L219 (-228.6977, 64.525) -> (-218.6977, 64.525)
  line L220 (-228.6977, 61.525) -> (-223.6977, 61.525)
  line L221 (-218.6977, 61.525) -> (-223.6977, 61.525)
  arc A144 (-208.6977, 64.525) -> (-208.6977, 61.525) centre (-208.6977, 63.025) ccw
  arc A145 (-198.6977, 61.525) -> (-198.6977, 64.525) centre (-198.6977, 63.025) ccw
  line L222 (-208.6977, 64.525) -> (-198.6977, 64.525)
  line L223 (-208.6977, 61.525) -> (-203.6977, 61.525)
  line L224 (-198.6977, 61.525) -> (-203.6977, 61.525)
  arc A146 (-188.6977, 64.525) -> (-188.6977, 61.525) centre (-188.6977, 63.025) ccw
  arc A147 (-178.6977, 61.525) -> (-178.6977, 64.525) centre (-178.6977, 63.025) ccw
  line L225 (-188.6977, 64.525) -> (-178.6977, 64.525)
  line L226 (-188.6977, 61.525) -> (-183.6977, 61.525)
  line L227 (-178.6977, 61.525) -> (-183.6977, 61.525)
  arc A148 (-168.6977, 64.525) -> (-168.6977, 61.525) centre (-168.6977, 63.025) ccw
  arc A149 (-158.6977, 61.525) -> (-158.6977, 64.525) centre (-158.6977, 63.025) ccw
  line L228 (-168.6977, 64.525) -> (-158.6977, 64.525)
  line L229 (-168.6977, 61.525) -> (-163.6977, 61.525)
  line L230 (-158.6977, 61.525) -> (-163.6977, 61.525)
  arc A150 (-148.6977, 64.525) -> (-148.6977, 61.525) centre (-148.6977, 63.025) ccw
  arc A151 (-138.6977, 61.525) -> (-138.6977, 64.525) centre (-138.6977, 63.025) ccw
  line L231 (-148.6977, 64.525) -> (-138.6977, 64.525)
  line L232 (-148.6977, 61.525) -> (-143.6977, 61.525)
  line L233 (-138.6977, 61.525) -> (-143.6977, 61.525)
  arc A152 (-128.6977, 64.525) -> (-128.6977, 61.525) centre (-128.6977, 63.025) ccw
  arc A153 (-118.6977, 61.525) -> (-118.6977, 64.525) centre (-118.6977, 63.025) ccw
  line L234 (-128.6977, 64.525) -> (-118.6977, 64.525)
  line L235 (-128.6977, 61.525) -> (-123.6977, 61.525)
  line L236 (-118.6977, 61.525) -> (-123.6977, 61.525)
  arc A154 (-108.6977, 64.525) -> (-108.6977, 61.525) centre (-108.6977, 63.025) ccw
  arc A155 (-98.6977, 61.525) -> (-98.6977, 64.525) centre (-98.6977, 63.025) ccw
  line L237 (-108.6977, 64.525) -> (-98.6977, 64.525)
  line L238 (-108.6977, 61.525) -> (-103.6977, 61.525)
  line L239 (-98.6977, 61.525) -> (-103.6977, 61.525)
  arc A156 (-88.6977, 64.525) -> (-88.6977, 61.525) centre (-88.6977, 63.025) ccw
  arc A157 (-78.6977, 61.525) -> (-78.6977, 64.525) centre (-78.6977, 63.025) ccw
  line L240 (-88.6977, 64.525) -> (-78.6977, 64.525)
  line L241 (-88.6977, 61.525) -> (-83.6977, 61.525)
  line L242 (-78.6977, 61.525) -> (-83.6977, 61.525)
  arc A158 (-68.6977, 64.525) -> (-68.6977, 61.525) centre (-68.6977, 63.025) ccw
  arc A159 (-58.6977, 61.525) -> (-58.6977, 64.525) centre (-58.6977, 63.025) ccw
  line L243 (-68.6977, 64.525) -> (-58.6977, 64.525)
  line L244 (-68.6977, 61.525) -> (-63.6977, 61.525)
  line L245 (-58.6977, 61.525) -> (-63.6977, 61.525)
  arc A160 (-248.6977, 74.525) -> (-248.6977, 71.525) centre (-248.6977, 73.025) ccw
  arc A161 (-238.6977, 71.525) -> (-238.6977, 74.525) centre (-238.6977, 73.025) ccw
  line L246 (-248.6977, 74.525) -> (-238.6977, 74.525)
  line L247 (-248.6977, 71.525) -> (-243.6977, 71.525)
  line L248 (-238.6977, 71.525) -> (-243.6977, 71.525)
  arc A162 (-228.6977, 74.525) -> (-228.6977, 71.525) centre (-228.6977, 73.025) ccw
  arc A163 (-218.6977, 71.525) -> (-218.6977, 74.525) centre (-218.6977, 73.025) ccw
  line L249 (-228.6977, 74.525) -> (-218.6977, 74.525)
  line L250 (-228.6977, 71.525) -> (-223.6977, 71.525)
  line L251 (-218.6977, 71.525) -> (-223.6977, 71.525)
  arc A164 (-208.6977, 74.525) -> (-208.6977, 71.525) centre (-208.6977, 73.025) ccw
  arc A165 (-198.6977, 71.525) -> (-198.6977, 74.525) centre (-198.6977, 73.025) ccw
  line L252 (-208.6977, 74.525) -> (-198.6977, 74.525)
  line L253 (-208.6977, 71.525) -> (-203.6977, 71.525)
  line L254 (-198.6977, 71.525) -> (-203.6977, 71.525)
  arc A166 (-188.6977, 74.525) -> (-188.6977, 71.525) centre (-188.6977, 73.025) ccw
  arc A167 (-178.6977, 71.525) -> (-178.6977, 74.525) centre (-178.6977, 73.025) ccw
  line L255 (-188.6977, 74.525) -> (-178.6977, 74.525)
  line L256 (-188.6977, 71.525) -> (-183.6977, 71.525)
  line L257 (-178.6977, 71.525) -> (-183.6977, 71.525)
  arc A168 (-168.6977, 74.525) -> (-168.6977, 71.525) centre (-168.6977, 73.025) ccw
  arc A169 (-158.6977, 71.525) -> (-158.6977, 74.525) centre (-158.6977, 73.025) ccw
  line L258 (-168.6977, 74.525) -> (-158.6977, 74.525)
  line L259 (-168.6977, 71.525) -> (-163.6977, 71.525)
  line L260 (-158.6977, 71.525) -> (-163.6977, 71.525)
  arc A170 (-128.6977, 74.525) -> (-128.6977, 71.525) centre (-128.6977, 73.025) ccw
  arc A171 (-118.6977, 71.525) -> (-118.6977, 74.525) centre (-118.6977, 73.025) ccw
  line L261 (-128.6977, 74.525) -> (-118.6977, 74.525)
  line L262 (-128.6977, 71.525) -> (-123.6977, 71.525)
  line L263 (-118.6977, 71.525) -> (-123.6977, 71.525)
  arc A172 (-108.6977, 74.525) -> (-108.6977, 71.525) centre (-108.6977, 73.025) ccw
  arc A173 (-98.6977, 71.525) -> (-98.6977, 74.525) centre (-98.6977, 73.025) ccw
  line L264 (-108.6977, 74.525) -> (-98.6977, 74.525)
  line L265 (-108.6977, 71.525) -> (-103.6977, 71.525)
  line L266 (-98.6977, 71.525) -> (-103.6977, 71.525)
  arc A174 (-88.6977, 74.525) -> (-88.6977, 71.525) centre (-88.6977, 73.025) ccw
  arc A175 (-78.6977, 71.525) -> (-78.6977, 74.525) centre (-78.6977, 73.025) ccw
  line L267 (-88.6977, 74.525) -> (-78.6977, 74.525)
  line L268 (-88.6977, 71.525) -> (-83.6977, 71.525)
  line L269 (-78.6977, 71.525) -> (-83.6977, 71.525)
  arc A176 (-68.6977, 74.525) -> (-68.6977, 71.525) centre (-68.6977, 73.025) ccw
  arc A177 (-58.6977, 71.525) -> (-58.6977, 74.525) centre (-58.6977, 73.025) ccw
  line L270 (-68.6977, 74.525) -> (-58.6977, 74.525)
  line L271 (-68.6977, 71.525) -> (-63.6977, 71.525)
  line L272 (-58.6977, 71.525) -> (-63.6977, 71.525)
  arc A178 (-248.6977, 84.525) -> (-248.6977, 81.525) centre (-248.6977, 83.025) ccw
  arc A179 (-238.6977, 81.525) -> (-238.6977, 84.525) centre (-238.6977, 83.025) ccw
  line L273 (-248.6977, 84.525) -> (-238.6977, 84.525)
  line L274 (-248.6977, 81.525) -> (-243.6977, 81.525)
  line L275 (-238.6977, 81.525) -> (-243.6977, 81.525)
  arc A180 (-228.6977, 84.525) -> (-228.6977, 81.525) centre (-228.6977, 83.025) ccw
  arc A181 (-218.6977, 81.525) -> (-218.6977, 84.525) centre (-218.6977, 83.025) ccw
  line L276 (-228.6977, 84.525) -> (-218.6977, 84.525)
  line L277 (-228.6977, 81.525) -> (-223.6977, 81.525)
  line L278 (-218.6977, 81.525) -> (-223.6977, 81.525)
  arc A182 (-208.6977, 84.525) -> (-208.6977, 81.525) centre (-208.6977, 83.025) ccw
  arc A183 (-198.6977, 81.525) -> (-198.6977, 84.525) centre (-198.6977, 83.025) ccw
  line L279 (-208.6977, 84.525) -> (-198.6977, 84.525)
  line L280 (-208.6977, 81.525) -> (-203.6977, 81.525)
  line L281 (-198.6977, 81.525) -> (-203.6977, 81.525)
  arc A184 (-188.6977, 84.525) -> (-188.6977, 81.525) centre (-188.6977, 83.025) ccw
  arc A185 (-178.6977, 81.525) -> (-178.6977, 84.525) centre (-178.6977, 83.025) ccw
  line L282 (-188.6977, 84.525) -> (-178.6977, 84.525)
  line L283 (-188.6977, 81.525) -> (-183.6977, 81.525)
  line L284 (-178.6977, 81.525) -> (-183.6977, 81.525)
  arc A186 (-168.6977, 84.525) -> (-168.6977, 81.525) centre (-168.6977, 83.025) ccw
  arc A187 (-158.6977, 81.525) -> (-158.6977, 84.525) centre (-158.6977, 83.025) ccw
  line L285 (-168.6977, 84.525) -> (-158.6977, 84.525)
  line L286 (-168.6977, 81.525) -> (-163.6977, 81.525)
  line L287 (-158.6977, 81.525) -> (-163.6977, 81.525)
  arc A188 (-148.6977, 84.525) -> (-148.6977, 81.525) centre (-148.6977, 83.025) ccw
  arc A189 (-138.6977, 81.525) -> (-138.6977, 84.525) centre (-138.6977, 83.025) ccw
  line L288 (-148.6977, 84.525) -> (-138.6977, 84.525)
  line L289 (-148.6977, 81.525) -> (-143.6977, 81.525)
  line L290 (-138.6977, 81.525) -> (-143.6977, 81.525)
  arc A190 (-128.6977, 84.525) -> (-128.6977, 81.525) centre (-128.6977, 83.025) ccw
  arc A191 (-118.6977, 81.525) -> (-118.6977, 84.525) centre (-118.6977, 83.025) ccw
  line L291 (-128.6977, 84.525) -> (-118.6977, 84.525)
  line L292 (-128.6977, 81.525) -> (-123.6977, 81.525)
  line L293 (-118.6977, 81.525) -> (-123.6977, 81.525)
  arc A192 (-108.6977, 84.525) -> (-108.6977, 81.525) centre (-108.6977, 83.025) ccw
  arc A193 (-98.6977, 81.525) -> (-98.6977, 84.525) centre (-98.6977, 83.025) ccw
  line L294 (-108.6977, 84.525) -> (-98.6977, 84.525)
  line L295 (-108.6977, 81.525) -> (-103.6977, 81.525)
  line L296 (-98.6977, 81.525) -> (-103.6977, 81.525)
  arc A194 (-88.6977, 84.525) -> (-88.6977, 81.525) centre (-88.6977, 83.025) ccw
  arc A195 (-78.6977, 81.525) -> (-78.6977, 84.525) centre (-78.6977, 83.025) ccw
  line L297 (-88.6977, 84.525) -> (-78.6977, 84.525)
  line L298 (-88.6977, 81.525) -> (-83.6977, 81.525)
  line L299 (-78.6977, 81.525) -> (-83.6977, 81.525)
  arc A196 (-68.6977, 84.525) -> (-68.6977, 81.525) centre (-68.6977, 83.025) ccw
  arc A197 (-58.6977, 81.525) -> (-58.6977, 84.525) centre (-58.6977, 83.025) ccw
  line L300 (-68.6977, 84.525) -> (-58.6977, 84.525)
  line L301 (-68.6977, 81.525) -> (-63.6977, 81.525)
  line L302 (-58.6977, 81.525) -> (-63.6977, 81.525)
  arc A198 (-248.6977, 94.525) -> (-248.6977, 91.525) centre (-248.6977, 93.025) ccw
  arc A199 (-238.6977, 91.525) -> (-238.6977, 94.525) centre (-238.6977, 93.025) ccw
  line L303 (-248.6977, 94.525) -> (-238.6977, 94.525)
  line L304 (-248.6977, 91.525) -> (-243.6977, 91.525)
  line L305 (-238.6977, 91.525) -> (-243.6977, 91.525)
  arc A200 (-228.6977, 94.525) -> (-228.6977, 91.525) centre (-228.6977, 93.025) ccw
  arc A201 (-218.6977, 91.525) -> (-218.6977, 94.525) centre (-218.6977, 93.025) ccw
  line L306 (-228.6977, 94.525) -> (-218.6977, 94.525)
  line L307 (-228.6977, 91.525) -> (-223.6977, 91.525)
  line L308 (-218.6977, 91.525) -> (-223.6977, 91.525)
  arc A202 (-208.6977, 94.525) -> (-208.6977, 91.525) centre (-208.6977, 93.025) ccw
  arc A203 (-198.6977, 91.525) -> (-198.6977, 94.525) centre (-198.6977, 93.025) ccw
  line L309 (-208.6977, 94.525) -> (-198.6977, 94.525)
  line L310 (-208.6977, 91.525) -> (-203.6977, 91.525)
  line L311 (-198.6977, 91.525) -> (-203.6977, 91.525)
  arc A204 (-188.6977, 94.525) -> (-188.6977, 91.525) centre (-188.6977, 93.025) ccw
  arc A205 (-178.6977, 91.525) -> (-178.6977, 94.525) centre (-178.6977, 93.025) ccw
  line L312 (-188.6977, 94.525) -> (-178.6977, 94.525)
  line L313 (-188.6977, 91.525) -> (-183.6977, 91.525)
  line L314 (-178.6977, 91.525) -> (-183.6977, 91.525)
  arc A206 (-168.6977, 94.525) -> (-168.6977, 91.525) centre (-168.6977, 93.025) ccw
  arc A207 (-158.6977, 91.525) -> (-158.6977, 94.525) centre (-158.6977, 93.025) ccw
  line L315 (-168.6977, 94.525) -> (-158.6977, 94.525)
  line L316 (-168.6977, 91.525) -> (-163.6977, 91.525)
  line L317 (-158.6977, 91.525) -> (-163.6977, 91.525)
  arc A208 (-148.6977, 94.525) -> (-148.6977, 91.525) centre (-148.6977, 93.025) ccw
  arc A209 (-138.6977, 91.525) -> (-138.6977, 94.525) centre (-138.6977, 93.025) ccw
  line L318 (-148.6977, 94.525) -> (-138.6977, 94.525)
  line L319 (-148.6977, 91.525) -> (-143.6977, 91.525)
  line L320 (-138.6977, 91.525) -> (-143.6977, 91.525)
  arc A210 (-128.6977, 94.525) -> (-128.6977, 91.525) centre (-128.6977, 93.025) ccw
  arc A211 (-118.6977, 91.525) -> (-118.6977, 94.525) centre (-118.6977, 93.025) ccw
  line L321 (-128.6977, 94.525) -> (-118.6977, 94.525)
  line L322 (-128.6977, 91.525) -> (-123.6977, 91.525)
  line L323 (-118.6977, 91.525) -> (-123.6977, 91.525)
  arc A212 (-108.6977, 94.525) -> (-108.6977, 91.525) centre (-108.6977, 93.025) ccw
  arc A213 (-98.6977, 91.525) -> (-98.6977, 94.525) centre (-98.6977, 93.025) ccw
  line L324 (-108.6977, 94.525) -> (-98.6977, 94.525)
  line L325 (-108.6977, 91.525) -> (-103.6977, 91.525)
  line L326 (-98.6977, 91.525) -> (-103.6977, 91.525)
  arc A214 (-88.6977, 94.525) -> (-88.6977, 91.525) centre (-88.6977, 93.025) ccw
  arc A215 (-78.6977, 91.525) -> (-78.6977, 94.525) centre (-78.6977, 93.025) ccw
  line L327 (-88.6977, 94.525) -> (-78.6977, 94.525)
  line L328 (-88.6977, 91.525) -> (-83.6977, 91.525)
  line L329 (-78.6977, 91.525) -> (-83.6977, 91.525)
  arc A216 (-68.6977, 94.525) -> (-68.6977, 91.525) centre (-68.6977, 93.025) ccw
  arc A217 (-58.6977, 91.525) -> (-58.6977, 94.525) centre (-58.6977, 93.025) ccw
  line L330 (-68.6977, 94.525) -> (-58.6977, 94.525)
  line L331 (-68.6977, 91.525) -> (-63.6977, 91.525)
  line L332 (-58.6977, 91.525) -> (-63.6977, 91.525)
  arc A218 (-248.6977, 104.525) -> (-248.6977, 101.525) centre (-248.6977, 103.025) ccw
  arc A219 (-238.6977, 101.525) -> (-238.6977, 104.525) centre (-238.6977, 103.025) ccw
  line L333 (-248.6977, 104.525) -> (-238.6977, 104.525)
  line L334 (-248.6977, 101.525) -> (-243.6977, 101.525)
  line L335 (-238.6977, 101.525) -> (-243.6977, 101.525)
  arc A220 (-228.6977, 104.525) -> (-228.6977, 101.525) centre (-228.6977, 103.025) ccw
  arc A221 (-218.6977, 101.525) -> (-218.6977, 104.525) centre (-218.6977, 103.025) ccw
  line L336 (-228.6977, 104.525) -> (-218.6977, 104.525)
  line L337 (-228.6977, 101.525) -> (-223.6977, 101.525)
  line L338 (-218.6977, 101.525) -> (-223.6977, 101.525)
  arc A222 (-208.6977, 104.525) -> (-208.6977, 101.525) centre (-208.6977, 103.025) ccw
  arc A223 (-198.6977, 101.525) -> (-198.6977, 104.525) centre (-198.6977, 103.025) ccw
  line L339 (-208.6977, 104.525) -> (-198.6977, 104.525)
  line L340 (-208.6977, 101.525) -> (-203.6977, 101.525)
  line L341 (-198.6977, 101.525) -> (-203.6977, 101.525)
  arc A224 (-188.6977, 104.525) -> (-188.6977, 101.525) centre (-188.6977, 103.025) ccw
  arc A225 (-178.6977, 101.525) -> (-178.6977, 104.525) centre (-178.6977, 103.025) ccw
  line L342 (-188.6977, 104.525) -> (-178.6977, 104.525)
  line L343 (-188.6977, 101.525) -> (-183.6977, 101.525)
  line L344 (-178.6977, 101.525) -> (-183.6977, 101.525)
  arc A226 (-168.6977, 104.525) -> (-168.6977, 101.525) centre (-168.6977, 103.025) ccw
  arc A227 (-158.6977, 101.525) -> (-158.6977, 104.525) centre (-158.6977, 103.025) ccw
  line L345 (-168.6977, 104.525) -> (-158.6977, 104.525)
  line L346 (-168.6977, 101.525) -> (-163.6977, 101.525)
  line L347 (-158.6977, 101.525) -> (-163.6977, 101.525)
  arc A228 (-148.6977, 104.525) -> (-148.6977, 101.525) centre (-148.6977, 103.025) ccw
  arc A229 (-138.6977, 101.525) -> (-138.6977, 104.525) centre (-138.6977, 103.025) ccw
  line L348 (-148.6977, 104.525) -> (-138.6977, 104.525)
  line L349 (-148.6977, 101.525) -> (-143.6977, 101.525)
  line L350 (-138.6977, 101.525) -> (-143.6977, 101.525)
  arc A230 (-128.6977, 104.525) -> (-128.6977, 101.525) centre (-128.6977, 103.025) ccw
  arc A231 (-118.6977, 101.525) -> (-118.6977, 104.525) centre (-118.6977, 103.025) ccw
  line L351 (-128.6977, 104.525) -> (-118.6977, 104.525)
  line L352 (-128.6977, 101.525) -> (-123.6977, 101.525)
  line L353 (-118.6977, 101.525) -> (-123.6977, 101.525)
  arc A232 (-108.6977, 104.525) -> (-108.6977, 101.525) centre (-108.6977, 103.025) ccw
  arc A233 (-98.6977, 101.525) -> (-98.6977, 104.525) centre (-98.6977, 103.025) ccw